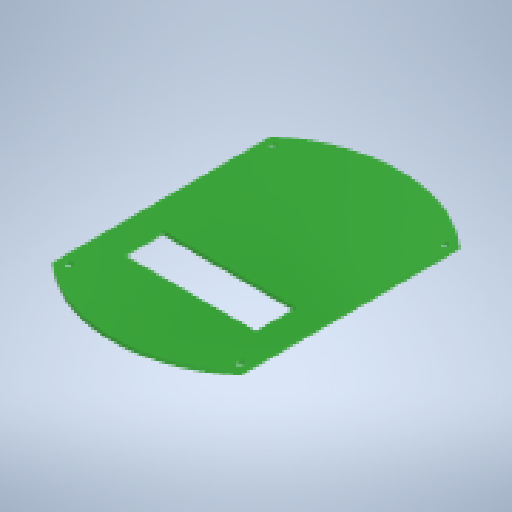
# Autodesk Inventor part: BaseBoard2
Saved by Autodesk Inventor 2025.3 (Build 293356000, 356)
## iProperties
Created: 2025-05-29
Part Number: BaseBoard2
Material: 一般
Document SubType Name: Modeling
Designer: yamashita1
Density: 1 g/cm^3
Appearance: 滑らか - 濃い深緑
Author: yamashita1
Autodesk Inventor part; units mm, degrees
ref_plane "YZ Plane" through (0, 0, 0) normal (1, 0, 0) x (0, 1, 0)
ref_plane "XZ Plane" through (0, 0, 0) normal (0, 1, 0) x (-1, 0, 0)
ref_plane "XY Plane" through (0, 0, 0) normal (0, 0, 1) x (1, 0, 0)
sketch "スケッチ1" plane through (0, 0, 0) normal (0, 0, 1) x (1, 0, 0)
  circle A0 centre (0, 0) radius 65 construction
  line L0 (-42.5, 65) -> (42.5, 65) construction
  line L1 (42.5, 65) -> (42.5, -65) construction
  line L2 (42.5, -65) -> (-42.5, -65) construction
  line L3 (-42.5, -65) -> (-42.5, 65) construction
  arc A1 (42.5, 49.1808) -> (-42.5, 49.1808) centre (0, 0) ccw
  line L4 (-42.5, 49.1808) -> (-42.5, -49.1808)
  line L5 (42.5, 49.1808) -> (42.5, -49.1808)
  arc A2 (-42.5, -49.1808) -> (42.5, -49.1808) centre (0, 0) ccw
  point P0 (0, 65)
  dimension "d0" = 130
  dimension "d1" = 85
  constraints: 14 end point, 9 point on circle, 4 point on line, 3 centre point, 3 parallel, 2 tangent, 1 coincident, 1 concentric, 1 horizontal, 1 midpoint, 1 perpendicular, 1 vertical, 1 vertical alignment
  measures "d0" diameter of A0
  measures "d1" distance of L1.end L2.end
extrude "基板" add sketch "スケッチ1" along normal blind 1.6
sketch "スケッチ4" plane through (0, 0, 1.6) normal (0, 0, 1) x (1, 0, 0)
  line L0 (0, -55.1622) -> (0, 55.1622) construction
  line L1 (42.5, -49.1808) -> (42.5, 49.1808) construction
  circle A0 centre (0, 0) radius 60 construction
  line L2 (0, 0) -> (36.3616, 43.334) construction
  line L3 (0, 0) -> (56.5685, 0) construction
  point P0 (38.5, -46.019)
  point P1 (-38.5, -46.019)
  point P2 (38.5673, 45.9627)
  point P3 (-38.5673, 45.9627)
  dimension "d27" = 4
  dimension "d29" = 120
  dimension "d30" = 50
  constraints: 6 end point, 2 coincident, 2 point on circle, 2 symmetric about line, 1 centre point, 1 equal length, 1 horizontal, 1 midpoint, 1 point on line, 1 vertical
  measures "d27" distance from line of L1 A0.end
  measures "d29" diameter of A0
  measures "d30" angle of L3 L2
hole "スペーサ取付穴" at (38.5, -46.019, 1.6) at (-38.5, -46.019, 1.6) at (38.5673, 45.9627, 1.6) at (-38.5673, 45.9627, 1.6) direction (0, 0, -1) diameter 3.2 end through all
sketch "スケッチ5" plane through (0, 0, 1.6) normal (0, 0, 1) x (1, 0, 0)
  line L0 (-30, -12) -> (30, -12)
  line L1 (30, -12) -> (30, -30)
  line L2 (30, -30) -> (-30, -30)
  line L3 (-30, -30) -> (-30, -12)
  point P0 (0, 0)
  point P1 (0, -12)
  dimension "d38" = 60
  dimension "d39" = 18
  dimension "d40" = 12
  constraints: 8 end point, 2 parallel, 1 horizontal, 1 midpoint, 1 perpendicular, 1 vertical alignment
  measures "d38" distance of L1.end L2.end
  measures "d39" distance of L0.end L1.end
  measures "d40" distance from line of L0 point (0, 0)
extrude "バッテリー通し穴" cut sketch "スケッチ5" against normal through all
